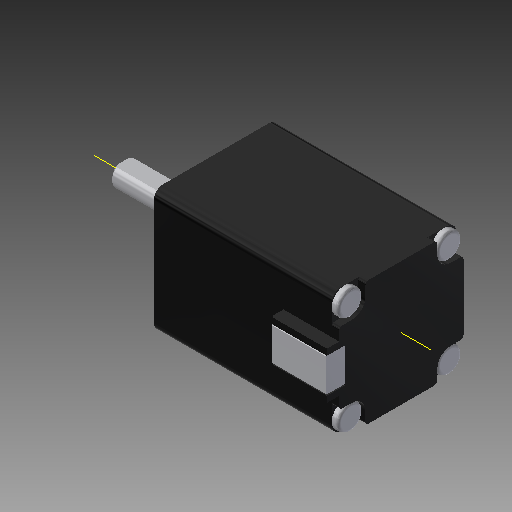
# Autodesk Inventor part: Stepper-motor-Nema-8
Saved by Autodesk Inventor 2019 (Build 230136000, 136)
## iProperties
Created: 2015-11-16
Part Number: Stepper-motor-Nema-8
Material: Generic
Document SubType Name: Modeling
Designer: Administrator
Density: 1 g/cm^3
Appearance: Default
Author: Administrator
Autodesk Inventor part; units mm, degrees
ref_plane "YZ Plane" through (0, 0, 0) normal (1, 0, 0) x (0, 1, 0)
ref_plane "XZ Plane" through (0, 0, 0) normal (0, 1, 0) x (-1, 0, 0)
ref_plane "XY Plane" through (0, 0, 0) normal (0, 0, 1) x (1, 0, 0)
sketch "Sketch1" plane through (0, 0, 0) normal (1, 0, 0) x (0, 1, 0)
  line L0 (-8.55, 10.05) -> (8.55, 10.05)
  line L1 (10.05, 8.55) -> (10.05, -8.55)
  line L2 (8.55, -10.05) -> (-8.55, -10.05)
  line L3 (-10.05, -8.55) -> (-10.05, 8.55)
  line L4 (-10.05, 10.05) -> (10.05, -10.05) construction
  line L5 (10.05, 10.05) -> (-10.05, -10.05) construction
  arc A0 (10.05, 8.55) -> (8.55, 10.05) centre (8.55, 8.55) ccw
  arc A1 (8.55, -10.05) -> (10.05, -8.55) centre (8.55, -8.55) ccw
  arc A2 (-10.05, -8.55) -> (-8.55, -10.05) centre (-8.55, -8.55) ccw
  arc A3 (-8.55, 10.05) -> (-10.05, 8.55) centre (-8.55, 8.55) ccw
  circle A4 centre (8, 8) radius 1.05 construction
  circle A5 centre (-8, 8) radius 1.05 construction
  circle A6 centre (-8, -8) radius 1.05 construction
  circle A7 centre (8, -8) radius 1.05 construction
  point P0 (0, 0)
  dimension "d2" = 20.1
  dimension "d3" = 20.1
  dimension "d4" = 1.5
  dimension "d5" = 2.1
  dimension "d6" = 8
  dimension "d9" = 360
  constraints: 12 end point, 9 point on line, 8 centre point, 8 point on circle, 8 tangent, 3 equal radius, 2 midpoint, 2 parallel, 1 horizontal, 1 perpendicular, 9 other
  measures "d2" distance of L4.end L5.end
  measures "d3" distance of L5.start L4.end
  measures "d4" radius of A0
  measures "d5" diameter of A4
  measures "d6" horizontal distance of A4.centre point (0, 0)
extrude "Extrusion3" add sketch "Sketch1" along normal blind 30
sketch "Sketch4" plane through (0, 0, 0) normal (-1, 0, 0) x (0, 0, 1)
  line L0 (8.55, 10.05) -> (-8.55, 10.05) projected
  arc A0 (-8.55, 10.05) -> (-10.05, 8.55) centre (-8.55, 8.55) ccw projected
  line L1 (-10.05, 8.55) -> (-10.05, -8.55) projected
  arc A1 (-10.05, -8.55) -> (-8.55, -10.05) centre (-8.55, -8.55) ccw projected
  line L2 (-8.55, -10.05) -> (8.55, -10.05) projected
  arc A2 (8.55, -10.05) -> (10.05, -8.55) centre (8.55, -8.55) ccw projected
  line L3 (10.05, -8.55) -> (10.05, 8.55) projected
  arc A3 (10.05, 8.55) -> (8.55, 10.05) centre (8.55, 8.55) ccw projected
  point P0 (0, 0)
  point P1 (-8, 8)
  point P2 (-8, -8)
  point P3 (8, -8)
  point P4 (8, 8)
hole "Hole1" at (0, 8, -8) at (0, -8, -8) at (0, -8, 8) at (0, 8, 8) direction (1, 0, 0) diameter 1.567 depth 3.5 tip angle 118 thread size "M2x0.4" class "6H" standard "ISO Metric profile"
chamfer "Chamfer1" distance 0.25 angle 45 4 edges at (0, 8, -8.7835) (0, 8, 7.2165) (0, -8, 7.2165) (0, -8, -8.7835)
sketch "Sketch5" plane through (0, 0, 0) normal (-1, 0, 0) x (0, 0, 1)
  circle A0 centre (0, 0) radius 7.5
  dimension "d27" = 15
  constraints: 1 centre point, 1 coincident
  measures "d27" diameter of A0
extrude "Extrusion4" add sketch "Sketch5" along normal blind 1.5
fillet "Fillet1" radius 0.15 2 edges at (0, 0, -7.5) (-1.5, 0, -7.5)
sketch "Sketch6" plane through (-1.5, 0, 0) normal (-1, 0, 0) x (0, 0, 1)
  circle A0 centre (0, 0) radius 2
  dimension "d31" = 4
  constraints: 1 centre point, 1 coincident
  measures "d31" diameter of A0
extrude "Extrusion5" add sketch "Sketch6" along normal blind 13.5
sketch "Sketch7" plane through (-15, 0, 0) normal (-1, 0, 0) x (0, 0, 1)
  circle A0 centre (0, 0) radius 2 projected
  line L0 (-1.3229, 1.5) -> (1.3229, 1.5)
  line L1 (0, 1.5) -> (0, -2) construction
  circle A1 centre (0, 0) radius 2 construction
  dimension "d35" = 3.5
  dimension "d36" = 90
  constraints: 4 end point, 3 point on circle, 1 horizontal, 1 midpoint, 1 vertical alignment, 1 other
  measures "d35" distance of L1.start L1.end
  measures "d36" angle of L1 L0
extrude "Extrusion6" cut sketch "Sketch7" against normal blind 12 contours L0 A0 picked at (-0.3089, 1.5908)
chamfer "Chamfer2" distance 0.25 angle 45 2 edges at (-15, -1.8229, -0.8229) (-15, 0.8229, 1.8229)
sketch "Sketch8" plane through (-1.5, 0, 0) normal (-1, 0, 0) x (0, 0, 1)
  circle A0 centre (0, 0) radius 2 projected
  circle A1 centre (0, 0) radius 4.5
  dimension "d42" = 9
  constraints: 1 centre point, 1 coincident
  measures "d42" diameter of A1
extrude "Extrusion7" cut sketch "Sketch8" against normal blind 0.5
chamfer "Chamfer3" distance 0.25 angle 45 1 edges at (-1, 0, -2)
sketch "Sketch9" plane through (30, 0, 0) normal (1, 0, 0) x (0, 0, -1)
  line L0 (8.55, 10.05) -> (-8.55, 10.05) projected
  arc A0 (-8.55, 10.05) -> (-10.05, 8.55) centre (-8.55, 8.55) ccw projected
  line L1 (-10.05, 8.55) -> (-10.05, -8.55) projected
  arc A1 (-10.05, -8.55) -> (-8.55, -10.05) centre (-8.55, -8.55) ccw projected
  line L2 (-8.55, -10.05) -> (8.55, -10.05) projected
  arc A2 (8.55, -10.05) -> (10.05, -8.55) centre (8.55, -8.55) ccw projected
  line L3 (10.05, -8.55) -> (10.05, 8.55) projected
  arc A3 (10.05, 8.55) -> (8.55, 10.05) centre (8.55, 8.55) ccw projected
  line L4 (8.55, 10.05) -> (-8.55, 10.05) projected
  line L5 (5.8, 10.05) -> (5.8, 8)
  line L6 (8, 5.8) -> (10.05, 5.8)
  line L7 (10.05, -8.55) -> (10.05, 8.55) projected
  circle A4 centre (-8, 8) radius 0.7835 projected
  circle A5 centre (-8, -8) radius 0.7835 projected
  circle A6 centre (8, -8) radius 0.7835 projected
  circle A7 centre (8, 8) radius 0.7835 projected
  circle A8 centre (8, 8) radius 2 construction
  arc A9 (5.8, 8) -> (8, 5.8) centre (8, 8) ccw
  point P0 (0, 0)
  dimension "d48" = 4
  dimension "d49" = 2.2
  dimension "d50" = 2.2
  dimension "d51" = 2.2
  constraints: 4 end point, 2 centre point, 2 point on circle, 2 point on line, 2 tangent, 1 coincident, 1 perpendicular, 1 vertical
  measures "d48" diameter of A8
  measures "d49" distance from line of L5 A7.centre
  measures "d50" distance from line of A7.centre L6
  measures "d51" radius of A9
extrude "Extrusion8" cut sketch "Sketch9" against normal blind 1.2 contours A3 L3 L6 A9 L5 L0 | A7
sketch "Sketch10" plane through (28.8, 0, 0) normal (1, 0, 0) x (0, 0, -1)
  circle A0 centre (8, 8) radius 2.05
  point P0 (0, 0)
  dimension "d55" = 4.1
  constraints: 1 centre point, 1 coincident
  measures "d55" diameter of A0
extrude "Extrusion9" add sketch "Sketch10" along normal blind 1
fillet "Fillet3" radius 0.5 1 edges at (29.8, 8, -5.95)
pattern_circular "Circular Pattern2" count 4 over 360 about axis through (-1.5, 0, 0) along (-1, 0, 0) of "Extrusion8", "Extrusion9", "Fillet3"
fillet "Fillet4" radius 0.5 8 edges at (29.4, 10.05, -5.8) (29.4, 5.8, -10.05) (29.4, -5.8, -10.05) (29.4, -10.05, -5.8) (29.4, -10.05, 5.8) (29.4, -5.8, 10.05) (29.4, 5.8, 10.05) (29.4, 10.05, 5.8)
sketch "Sketch12" plane through (0, -8.55, 10.05) normal (0, 0, 1) x (1, 0, 0)
  line L0 (30, 13.85) -> (30, 3.25) projected
  line L1 (39, 8.55) -> (-24, 8.55) projected
  line L2 (30, 3.25) -> (30, 13.85) projected
  line L3 (30, 12.35) -> (21, 12.35)
  line L4 (21, 12.35) -> (21, 11.35)
  line L5 (21, 11.35) -> (30, 11.35)
  line L6 (30, 11.35) -> (30, 12.35)
  line L7 (30, 4.75) -> (21, 4.75)
  line L8 (21, 4.75) -> (21, 5.75)
  line L9 (21, 5.75) -> (30, 5.75)
  line L10 (30, 5.75) -> (30, 4.75)
  point P0 (0, 8.55)
  dimension "d66" = 9
  dimension "d67" = 1
  dimension "d68" = 2.8
  constraints: 16 end point, 4 symmetric about line, 2 parallel, 1 horizontal, 1 perpendicular, 1 point on line
  measures "d66" distance of L5.end L4.end
  measures "d67" distance between parallel lines of L5 L3
  measures "d68" distance between parallel lines of L1 L5
extrude "Extrusion10" add sketch "Sketch12" along normal blind 2
chamfer "Chamfer4" distance 0.25 angle 45 2 edges at (21, 3.3, 12.05) (21, -3.3, 12.05)
sketch "Sketch13" plane through (30, 0, 0) normal (1, 0, 0) x (0, 0, -1)
  arc A0 (-5.3, 10.05) -> (-5.8, 9.55) centre (-5.3, 9.55) ccw projected
  line L0 (-5.8, 9.55) -> (-5.8, 8) projected
  arc A1 (-8, 5.8) -> (-5.8, 8) centre (-8, 8) ccw projected
  line L1 (-8, 5.8) -> (-9.55, 5.8) projected
  arc A2 (-9.55, 5.8) -> (-10.05, 5.3) centre (-9.55, 5.3) ccw projected
  line L2 (-10.05, 5.3) -> (-10.05, 3.8) projected
  line L3 (-10.05, 3.8) -> (-12.05, 3.8) projected
  line L4 (-12.05, 2.8) -> (-12.05, 3.8) projected
  line L5 (-10.05, 2.8) -> (-12.05, 2.8) projected
  line L6 (-10.05, 2.8) -> (-10.05, -2.8) projected
  line L7 (-10.05, -2.8) -> (-12.05, -2.8) projected
  line L8 (-12.05, -3.8) -> (-12.05, -2.8) projected
  line L9 (-10.05, -3.8) -> (-12.05, -3.8) projected
  line L10 (-10.05, -3.8) -> (-10.05, -5.3) projected
  arc A3 (-10.05, -5.3) -> (-9.55, -5.8) centre (-9.55, -5.3) ccw projected
  line L11 (-9.55, -5.8) -> (-8, -5.8) projected
  arc A4 (-5.8, -8) -> (-8, -5.8) centre (-8, -8) ccw projected
  line L12 (-5.8, -8) -> (-5.8, -9.55) projected
  arc A5 (-5.8, -9.55) -> (-5.3, -10.05) centre (-5.3, -9.55) ccw projected
  line L13 (-5.3, -10.05) -> (5.3, -10.05) projected
  arc A6 (5.3, -10.05) -> (5.8, -9.55) centre (5.3, -9.55) ccw projected
  line L14 (5.8, -9.55) -> (5.8, -8) projected
  arc A7 (8, -5.8) -> (5.8, -8) centre (8, -8) ccw projected
  line L15 (8, -5.8) -> (9.55, -5.8) projected
  arc A8 (9.55, -5.8) -> (10.05, -5.3) centre (9.55, -5.3) ccw projected
  line L16 (10.05, -5.3) -> (10.05, 5.3) projected
  arc A9 (10.05, 5.3) -> (9.55, 5.8) centre (9.55, 5.3) ccw projected
  line L17 (9.55, 5.8) -> (8, 5.8) projected
  arc A10 (5.8, 8) -> (8, 5.8) centre (8, 8) ccw projected
  line L18 (5.8, 8) -> (5.8, 9.55) projected
  arc A11 (5.8, 9.55) -> (5.3, 10.05) centre (5.3, 9.55) ccw projected
  line L19 (5.3, 10.05) -> (-5.3, 10.05) projected
  line L20 (-10.05, -2.8) -> (-9.05, -2.8)
  line L21 (-9.05, -2.8) -> (-9.05, 2.8)
  line L22 (-9.05, 2.8) -> (-10.05, 2.8)
  point P0 (0, 0)
  dimension "d74" = 1
  constraints: 6 end point, 2 perpendicular, 1 horizontal
  measures "d74" distance between parallel lines of L6 L21
extrude "Extrusion11" cut sketch "Sketch13" against normal up to surface (9 mm away) contours L22 L21 L20 L6
sketch "Sketch14" plane through (30, 0, 0) normal (1, 0, 0) x (0, 0, -1)
  line L0 (-9.05, 2.8) -> (-9.05, -2.8) projected
  line L1 (-9.05, -2.7) -> (-12.05, -2.7)
  line L2 (-12.05, -2.7) -> (-12.05, 2.7)
  line L3 (-12.05, 2.7) -> (-9.05, 2.7)
  line L4 (-9.05, 2.7) -> (-9.05, -2.7)
  line L5 (-12.05, 2.8) -> (-9.05, 2.8) projected
  line L6 (-9.05, 2.8) -> (-9.05, -2.8) projected
  line L7 (-9.05, -2.8) -> (-12.05, -2.8) projected
  line L8 (-12.05, -3.8) -> (-12.05, -2.8) projected
  line L9 (-10.05, -3.8) -> (-12.05, -3.8) projected
  line L10 (-10.05, -3.8) -> (-10.05, -5.3) projected
  arc A0 (-10.05, -5.3) -> (-9.55, -5.8) centre (-9.55, -5.3) ccw projected
  line L11 (-9.55, -5.8) -> (-8, -5.8) projected
  arc A1 (-5.8, -8) -> (-8, -5.8) centre (-8, -8) ccw projected
  line L12 (-5.8, -8) -> (-5.8, -9.55) projected
  arc A2 (-5.8, -9.55) -> (-5.3, -10.05) centre (-5.3, -9.55) ccw projected
  line L13 (-5.3, -10.05) -> (5.3, -10.05) projected
  arc A3 (5.3, -10.05) -> (5.8, -9.55) centre (5.3, -9.55) ccw projected
  line L14 (5.8, -9.55) -> (5.8, -8) projected
  arc A4 (8, -5.8) -> (5.8, -8) centre (8, -8) ccw projected
  line L15 (8, -5.8) -> (9.55, -5.8) projected
  arc A5 (9.55, -5.8) -> (10.05, -5.3) centre (9.55, -5.3) ccw projected
  line L16 (10.05, -5.3) -> (10.05, 5.3) projected
  arc A6 (10.05, 5.3) -> (9.55, 5.8) centre (9.55, 5.3) ccw projected
  line L17 (9.55, 5.8) -> (8, 5.8) projected
  arc A7 (5.8, 8) -> (8, 5.8) centre (8, 8) ccw projected
  line L18 (5.8, 8) -> (5.8, 9.55) projected
  arc A8 (5.8, 9.55) -> (5.3, 10.05) centre (5.3, 9.55) ccw projected
  line L19 (5.3, 10.05) -> (-5.3, 10.05) projected
  arc A9 (-5.3, 10.05) -> (-5.8, 9.55) centre (-5.3, 9.55) ccw projected
  line L20 (-5.8, 9.55) -> (-5.8, 8) projected
  arc A10 (-8, 5.8) -> (-5.8, 8) centre (-8, 8) ccw projected
  line L21 (-8, 5.8) -> (-9.55, 5.8) projected
  arc A11 (-9.55, 5.8) -> (-10.05, 5.3) centre (-9.55, 5.3) ccw projected
  line L22 (-10.05, 5.3) -> (-10.05, 3.8) projected
  line L23 (-10.05, 3.8) -> (-12.05, 3.8) projected
  line L24 (-12.05, 2.8) -> (-12.05, 3.8) projected
  line L25 (-12.05, 2.8) -> (-12.05, 3.8) projected
  point P0 (0, 0)
  dimension "d77" = 0.1
  dimension "d79" = 0.1
  constraints: 8 end point, 2 parallel, 1 collinear, 1 horizontal, 1 perpendicular, 1 point on line
  measures "d77" distance between parallel lines of L1 L7
  measures "d79" distance between parallel lines of L5 L3
extrude "Extrusion12" add sketch "Sketch14" against normal blind 8.95 contours L0 L1 L2 L3
fillet "Fillet5" radius 0.1 5 edges at (21.05, 2.7, 10.55) (21.05, 0, 12.05) (21.05, -2.7, 10.55) (25.525, -2.7, 12.05) (25.525, 2.7, 12.05)
sketch "Sketch15" plane through (30, 0, 0) normal (1, 0, 0) x (0, 0, -1)
  arc A0 (-11.95, 2.7) -> (-12.05, 2.6) centre (-11.95, 2.6) ccw projected
  line L0 (-12.05, -2.6) -> (-12.05, 2.6) projected
  arc A1 (-12.05, -2.6) -> (-11.95, -2.7) centre (-11.95, -2.6) ccw projected
  line L1 (-9.05, -2.7) -> (-11.95, -2.7) projected
  line L2 (-9.05, -2.7) -> (-9.05, -2.8) projected
  line L3 (-9.05, -2.8) -> (-12.05, -2.8) projected
  line L4 (-12.05, -3.8) -> (-12.05, -2.8) projected
  line L5 (-10.05, -3.8) -> (-12.05, -3.8) projected
  line L6 (-10.05, -3.8) -> (-10.05, -5.3) projected
  arc A2 (-10.05, -5.3) -> (-9.55, -5.8) centre (-9.55, -5.3) ccw projected
  line L7 (-9.55, -5.8) -> (-8, -5.8) projected
  arc A3 (-5.8, -8) -> (-8, -5.8) centre (-8, -8) ccw projected
  line L8 (-5.8, -8) -> (-5.8, -9.55) projected
  arc A4 (-5.8, -9.55) -> (-5.3, -10.05) centre (-5.3, -9.55) ccw projected
  line L9 (-5.3, -10.05) -> (5.3, -10.05) projected
  arc A5 (5.3, -10.05) -> (5.8, -9.55) centre (5.3, -9.55) ccw projected
  line L10 (5.8, -9.55) -> (5.8, -8) projected
  arc A6 (8, -5.8) -> (5.8, -8) centre (8, -8) ccw projected
  line L11 (8, -5.8) -> (9.55, -5.8) projected
  arc A7 (9.55, -5.8) -> (10.05, -5.3) centre (9.55, -5.3) ccw projected
  line L12 (10.05, -5.3) -> (10.05, 5.3) projected
  arc A8 (10.05, 5.3) -> (9.55, 5.8) centre (9.55, 5.3) ccw projected
  line L13 (9.55, 5.8) -> (8, 5.8) projected
  arc A9 (5.8, 8) -> (8, 5.8) centre (8, 8) ccw projected
  line L14 (5.8, 8) -> (5.8, 9.55) projected
  arc A10 (5.8, 9.55) -> (5.3, 10.05) centre (5.3, 9.55) ccw projected
  line L15 (5.3, 10.05) -> (-5.3, 10.05) projected
  arc A11 (-5.3, 10.05) -> (-5.8, 9.55) centre (-5.3, 9.55) ccw projected
  line L16 (-5.8, 9.55) -> (-5.8, 8) projected
  arc A12 (-8, 5.8) -> (-5.8, 8) centre (-8, 8) ccw projected
  line L17 (-8, 5.8) -> (-9.55, 5.8) projected
  arc A13 (-9.55, 5.8) -> (-10.05, 5.3) centre (-9.55, 5.3) ccw projected
  line L18 (-10.05, 5.3) -> (-10.05, 3.8) projected
  line L19 (-10.05, 3.8) -> (-12.05, 3.8) projected
  line L20 (-12.05, 2.8) -> (-12.05, 3.8) projected
  line L21 (-12.05, 2.8) -> (-9.05, 2.8) projected
  line L22 (-9.05, 2.8) -> (-9.05, 2.7) projected
  line L23 (-11.95, 2.7) -> (-9.05, 2.7) projected
  line L24 (-9.05, 2.7) -> (-9.05, -2.7)
  point P0 (0, 0)
  constraints: 2 end point, 1 vertical
extrude "Extrusion13" cut sketch "Sketch15" against normal blind 0.1 contours L23 L24 L1 A1 L0 A0
body "Solid2"
